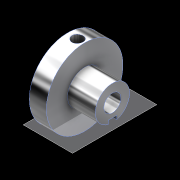
# Autodesk Inventor part: StepperAdapter
Saved by Autodesk Inventor 2018 (Build 220112000, 112)
## iProperties
Created: 2022-02-18
Part Number: StepperAdapter
Material: Aluminum 6061
Document SubType Name: Modeling
Designer: kumpu
Density: 2.7 g/cm^3
Appearance: Aluminum - Flat
Author: kumpu
Autodesk Inventor part; units mm, degrees
ref_plane "YZ Plane" through (0, 0, 0) normal (1, 0, 0) x (0, 1, 0)
ref_plane "XY Plane" through (0, 0, 0) normal (0, 0, 1) x (1, 0, 0)
sketch "Sketch1" plane through (0, 0, 0) normal (0, 1, 0) x (-1, 0, 0)
  line L0 (0, 0) -> (-16.637, 0)
  line L1 (0, 3.175) -> (-16.637, 3.175)
  line L2 (-16.637, 3.175) -> (-16.637, 6.35)
  line L3 (-16.637, 6.35) -> (-6.35, 6.35)
  line L4 (-6.35, 6.35) -> (-6.35, 14.224)
  line L5 (-6.35, 14.224) -> (0, 14.224)
  line L6 (0, 14.224) -> (0, 3.175)
  dimension "d0" = 12.7
  dimension "d1" = 6.35
  dimension "d2" = 10.287
  dimension "d4" = 28.448
  dimension "d5" = 6.35
  constraints: 14 end point, 5 perpendicular, 2 horizontal, 2 point on line
  measures "d0" diameter of L3 L0
  measures "d1" diameter of L1 L0
  measures "d2" distance of L2.end L3.end
  measures "d4" diameter of L5 L0
  measures "d5" distance of L4.end L5.end
revolve "Revolution1" add sketch "Sketch1" angle 360 about axis through (0, 0, 0) along (1, 0, 0)
sketch "Sketch2" plane through (0, 0, 0) normal (0, 1, 0) x (-1, 0, 0)
  circle A0 centre (-3.7338, 0) radius 2.0828
  line L0 (-3.7338, 0) -> (-16.637, 0) construction
  line L1 (-16.637, -3.175) -> (-16.637, 3.175) projected
  line L2 (-1.651, -4.0967) -> (-1.651, 3.8062) construction
  point P0 (0, 0)
  dimension "d7" = 4.1656
  dimension "d8" = 14.986
  constraints: 4 end point, 1 centre point, 1 horizontal, 1 midpoint, 1 tangent, 1 vertical
  measures "d7" diameter of A0
  measures "d8" distance between parallel lines of L1 L2
extrude "Extrusion1" cut sketch "Sketch2" along normal blind 25.4
ref_plane "Work Plane1" through (0, -7.9502, 0) normal (0, 1, 0) x (-1, 0, 0)
sketch "Sketch3" plane through (0, -7.9502, 0) normal (0, 1, 0) x (-1, 0, 0)
  line L0 (-7.9375, 0) -> (-16.637, 0) construction
  line L1 (-7.9375, 1.5875) -> (-16.637, 1.5875)
  line L2 (-16.637, -1.5875) -> (-7.9375, -1.5875)
  arc A0 (-7.9375, -1.5875) -> (-7.9375, 1.5875) centre (-7.9375, 0) ccw
  arc A1 (-16.637, 1.5875) -> (-16.637, -1.5875) centre (-16.637, 0) ccw
  line L3 (-6.35, -14.224) -> (-6.35, 14.224) projected
  line L4 (-16.637, -6.35) -> (-16.637, 6.35) projected
  point P0 (0, 0)
  point P1 (-12.2873, 0)
  dimension "d12" = 1.5875
  constraints: 8 end point, 5 tangent, 4 point on circle, 2 centre point, 2 point on line, 1 horizontal, 1 midpoint, 1 parallel
  measures "d12" radius of A1
extrude "Extrusion2" cut sketch "Sketch3" along normal blind 3.1496
body "Solid1"
